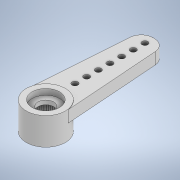
# Autodesk Inventor part: Серво-насадка односторонняя
Saved by Autodesk Inventor 2020 (Build 240168000, 168)
## iProperties
Created: 2021-04-04
Part Number: Серво-насадка односторонняя
Material: Типовые
Document SubType Name: Modeling
Designer: Антон
Density: 1 g/cm^3
Appearance: По умолчанию
Author: Антон
Autodesk Inventor part; units mm, degrees
ref_plane "YZ Plane" through (0, 0, 0) normal (1, 0, 0) x (0, 1, 0)
ref_plane "XZ Plane" through (0, 0, 0) normal (0, 1, 0) x (-1, 0, 0)
ref_plane "XY Plane" through (0, 0, 0) normal (0, 0, 1) x (1, 0, 0)
sketch "Эскиз1" plane through (0, 0, 0) normal (0, 1, 0) x (-1, 0, 0)
  circle A0 centre (0, 0) radius 3.35
  dimension "d0" = 6.7
  constraints: 1 centre point, 1 coincident
  measures "d0" diameter of A0
extrude "Выдавливание1" add sketch "Эскиз1" along normal blind 4.7
ref_plane "РабПлоскость1" through (0, 4.6, 0) normal (0, 1, 0) x (1, 0, 0)
sketch "Эскиз2" plane through (0, 4.6, 0) normal (0, 1, 0) x (1, 0, 0)
  circle A0 centre (0, 0) radius 3.35 projected
  circle A1 centre (0, 0) radius 3.35 projected
  line L0 (-3.35, 0) -> (3.35, 0)
  line L1 (3.35, 0) -> (3.35, 18.5)
  line L2 (3.35, 18.5) -> (-3.35, 18.5)
  line L3 (-3.35, 18.5) -> (-3.35, 0)
  line L4 (2, 0) -> (2, 18.5)
  line L5 (2, 18.5) -> (-2, 18.5)
  line L6 (-2, 18.5) -> (-2, 0)
  line L7 (-2, 0) -> (2, 0)
  line L8 (2, 0) -> (-2, 18.5) construction
  line L9 (2, 18.5) -> (-2, 0) construction
  line L10 (-3.35, 0) -> (-2, 18.5)
  line L11 (3.35, 0) -> (2, 18.5)
  point P0 (0, 9.25)
  point P1 (-3.3145, 0.4863)
  point P2 (3.3145, 0.4863)
  dimension "d4" = 18.5
  dimension "d5" = 4
  constraints: 24 end point, 4 parallel, 2 midpoint, 2 perpendicular, 1 horizontal, 1 horizontal alignment, 1 other
  measures "d4" distance of L1.end L0.end
  measures "d5" distance of L5.end L4.end
extrude "Выдавливание2" add sketch "Эскиз2" against normal blind 2 contours L10 L6 A0 | A0 L4 L11 | L6 L2 L4 A0
sketch "Эскиз3" plane through (0, 4.6, 0) normal (0, 1, 0) x (1, 0, 0)
  line L0 (-2, 18.5) -> (2, 18.5) projected
  line L1 (0, 18.5) -> (0, 17)
  circle A0 centre (0, 17) radius 0.5
  circle A1 centre (0, 15) radius 0.5
  circle A2 centre (0, 13) radius 0.5
  circle A3 centre (0, 11) radius 0.5
  circle A4 centre (0, 9) radius 0.5
  circle A5 centre (0, 7) radius 0.5
  circle A6 centre (0, 5) radius 0.5
  point P0 (0, 0)
  dimension "d8" = 1.5
  dimension "d9" = 1
  dimension "d12" = 2
  constraints: 7 centre point, 2 end point, 2 vertical, 1 coincident, 1 midpoint, 12 other
  measures "d8" distance of L1.start L1.end
  measures "d9" diameter of A0
  measures "d12" distance of A0.centre A1.centre
extrude "Выдавливание3" cut sketch "Эскиз3" against normal through all
fillet "Сопряжение1" radius 2 2 edges at (-2, 3.6, -18.5) (2, 3.6, -18.5)
sketch "Эскиз5" plane through (0, 4.7, 0) normal (0, 1, 0) x (1, 0, 0)
  point P0 (0, 0)
  point P1 (0, 0)
  constraints: 1 coincident
hole "Отверстие1" at (0, 4.7, 0) direction (0, -1, 0) diameter 2.7 end through all counterbore diameter 4.7 counterbore depth 1
sketch "Эскиз6" plane through (0, 0, 0) normal (0, -1, 0) x (1, 0, 0)
  circle A0 centre (0, 0) radius 1.35 projected
  circle A1 centre (0, 0) radius 3.35 projected
  line L0 (0, 0) -> (-2.375, 0)
  line L1 (-2.375, 0) -> (-2.4726, 0.0976)
  line L2 (-2.4726, 0.0976) -> (-2.4692, 0.1615)
  line L3 (-2.375, 0) -> (-2.4726, -0.0976)
  line L4 (-2.362, -0.2483) -> (-2.4692, -0.1614)
  line L5 (-2.4692, -0.1614) -> (-2.4726, -0.0975)
  line L6 (-2.362, -0.2483) -> (-2.4488, -0.3555)
  line L7 (-2.3231, -0.4938) -> (-2.4388, -0.4186)
  line L8 (-2.4388, -0.4186) -> (-2.4488, -0.3554)
  line L9 (-2.3231, -0.4938) -> (-2.3983, -0.6095)
  line L10 (-2.2588, -0.7339) -> (-2.3817, -0.6713)
  line L11 (-2.3817, -0.6713) -> (-2.3983, -0.6094)
  line L12 (-2.2588, -0.7339) -> (-2.3214, -0.8569)
  line L13 (-2.1697, -0.966) -> (-2.2985, -0.9165)
  line L14 (-2.2985, -0.9165) -> (-2.3214, -0.8568)
  line L15 (-2.1697, -0.966) -> (-2.2191, -1.0948)
  line L16 (-2.0568, -1.1875) -> (-2.1901, -1.1518)
  line L17 (-2.1901, -1.1518) -> (-2.2192, -1.0948)
  line L18 (-2.0568, -1.1875) -> (-2.0925, -1.3208)
  line L19 (-1.9214, -1.396) -> (-2.0577, -1.3744)
  line L20 (-2.0577, -1.3744) -> (-2.0926, -1.3207)
  line L21 (-1.9214, -1.396) -> (-1.943, -1.5323)
  line L22 (-1.765, -1.5892) -> (-1.9028, -1.582)
  line L23 (-1.9028, -1.582) -> (-1.9431, -1.5322)
  line L24 (-1.765, -1.5892) -> (-1.7722, -1.727)
  line L25 (-1.5892, -1.765) -> (-1.727, -1.7722)
  line L26 (-1.727, -1.7722) -> (-1.7723, -1.7269)
  line L27 (-1.5892, -1.765) -> (-1.582, -1.9028)
  line L28 (-1.396, -1.9214) -> (-1.5323, -1.943)
  line L29 (-1.5323, -1.943) -> (-1.582, -1.9027)
  line L30 (-1.396, -1.9214) -> (-1.3744, -2.0577)
  line L31 (-1.1875, -2.0568) -> (-1.3208, -2.0925)
  line L32 (-1.3208, -2.0925) -> (-1.3745, -2.0577)
  line L33 (-1.1875, -2.0568) -> (-1.1518, -2.1901)
  line L34 (-0.966, -2.1697) -> (-1.0948, -2.2191)
  line L35 (-1.0948, -2.2191) -> (-1.1519, -2.1901)
  line L36 (-0.966, -2.1697) -> (-0.9165, -2.2985)
  line L37 (-0.7339, -2.2588) -> (-0.8569, -2.3214)
  line L38 (-0.8569, -2.3214) -> (-0.9166, -2.2985)
  line L39 (-0.7339, -2.2588) -> (-0.6713, -2.3817)
  line L40 (-0.4938, -2.3231) -> (-0.6095, -2.3983)
  line L41 (-0.6095, -2.3983) -> (-0.6713, -2.3817)
  line L42 (-0.4938, -2.3231) -> (-0.4186, -2.4388)
  line L43 (-0.2483, -2.362) -> (-0.3555, -2.4488)
  line L44 (-0.3555, -2.4488) -> (-0.4187, -2.4388)
  line L45 (-0.2483, -2.362) -> (-0.1614, -2.4692)
  line L46 (0, -2.375) -> (-0.0976, -2.4726)
  line L47 (-0.0976, -2.4726) -> (-0.1615, -2.4692)
  line L48 (0, -2.375) -> (0.0976, -2.4726)
  line L49 (0.2483, -2.362) -> (0.1614, -2.4692)
  line L50 (0.1614, -2.4692) -> (0.0975, -2.4726)
  line L51 (0.2483, -2.362) -> (0.3555, -2.4488)
  line L52 (0.4938, -2.3231) -> (0.4186, -2.4388)
  line L53 (0.4186, -2.4388) -> (0.3554, -2.4488)
  line L54 (0.4938, -2.3231) -> (0.6095, -2.3983)
  line L55 (0.7339, -2.2588) -> (0.6713, -2.3817)
  line L56 (0.6713, -2.3817) -> (0.6094, -2.3983)
  line L57 (0.7339, -2.2588) -> (0.8569, -2.3214)
  line L58 (0.966, -2.1697) -> (0.9165, -2.2985)
  line L59 (0.9165, -2.2985) -> (0.8568, -2.3214)
  line L60 (0.966, -2.1697) -> (1.0948, -2.2191)
  line L61 (1.1875, -2.0568) -> (1.1518, -2.1901)
  line L62 (1.1518, -2.1901) -> (1.0948, -2.2192)
  line L63 (1.1875, -2.0568) -> (1.3208, -2.0925)
  line L64 (1.396, -1.9214) -> (1.3744, -2.0577)
  line L65 (1.3744, -2.0577) -> (1.3207, -2.0926)
  line L66 (1.396, -1.9214) -> (1.5323, -1.943)
  line L67 (1.5892, -1.765) -> (1.582, -1.9028)
  line L68 (1.582, -1.9028) -> (1.5322, -1.9431)
  line L69 (1.5892, -1.765) -> (1.727, -1.7722)
  line L70 (1.765, -1.5892) -> (1.7722, -1.727)
  line L71 (1.7722, -1.727) -> (1.7269, -1.7723)
  line L72 (1.765, -1.5892) -> (1.9028, -1.582)
  line L73 (1.9214, -1.396) -> (1.943, -1.5323)
  line L74 (1.943, -1.5323) -> (1.9027, -1.582)
  line L75 (1.9214, -1.396) -> (2.0577, -1.3744)
  line L76 (2.0568, -1.1875) -> (2.0925, -1.3208)
  line L77 (2.0925, -1.3208) -> (2.0577, -1.3745)
  line L78 (2.0568, -1.1875) -> (2.1901, -1.1518)
  line L79 (2.1697, -0.966) -> (2.2191, -1.0948)
  line L80 (2.2191, -1.0948) -> (2.1901, -1.1519)
  line L81 (2.1697, -0.966) -> (2.2985, -0.9165)
  line L82 (2.2588, -0.7339) -> (2.3214, -0.8569)
  line L83 (2.3214, -0.8569) -> (2.2985, -0.9166)
  line L84 (2.2588, -0.7339) -> (2.3817, -0.6713)
  line L85 (2.3231, -0.4938) -> (2.3983, -0.6095)
  line L86 (2.3983, -0.6095) -> (2.3817, -0.6713)
  line L87 (2.3231, -0.4938) -> (2.4388, -0.4186)
  line L88 (2.362, -0.2483) -> (2.4488, -0.3555)
  line L89 (2.4488, -0.3555) -> (2.4388, -0.4187)
  line L90 (2.362, -0.2483) -> (2.4692, -0.1614)
  line L91 (2.375, 0) -> (2.4726, -0.0976)
  line L92 (2.4726, -0.0976) -> (2.4692, -0.1615)
  line L93 (2.375, 0) -> (2.4726, 0.0976)
  line L94 (2.362, 0.2483) -> (2.4692, 0.1614)
  line L95 (2.4692, 0.1614) -> (2.4726, 0.0975)
  line L96 (2.362, 0.2483) -> (2.4488, 0.3555)
  line L97 (2.3231, 0.4938) -> (2.4388, 0.4186)
  line L98 (2.4388, 0.4186) -> (2.4488, 0.3554)
  line L99 (2.3231, 0.4938) -> (2.3983, 0.6095)
  line L100 (2.2588, 0.7339) -> (2.3817, 0.6713)
  line L101 (2.3817, 0.6713) -> (2.3983, 0.6094)
  line L102 (2.2588, 0.7339) -> (2.3214, 0.8569)
  line L103 (2.1697, 0.966) -> (2.2985, 0.9165)
  line L104 (2.2985, 0.9165) -> (2.3214, 0.8568)
  line L105 (2.1697, 0.966) -> (2.2191, 1.0948)
  line L106 (2.0568, 1.1875) -> (2.1901, 1.1518)
  line L107 (2.1901, 1.1518) -> (2.2192, 1.0948)
  line L108 (2.0568, 1.1875) -> (2.0925, 1.3208)
  line L109 (1.9214, 1.396) -> (2.0577, 1.3744)
  line L110 (2.0577, 1.3744) -> (2.0926, 1.3207)
  line L111 (1.9214, 1.396) -> (1.943, 1.5323)
  line L112 (1.765, 1.5892) -> (1.9028, 1.582)
  line L113 (1.9028, 1.582) -> (1.9431, 1.5322)
  line L114 (1.765, 1.5892) -> (1.7722, 1.727)
  line L115 (1.5892, 1.765) -> (1.727, 1.7722)
  line L116 (1.727, 1.7722) -> (1.7723, 1.7269)
  line L117 (1.5892, 1.765) -> (1.582, 1.9028)
  line L118 (1.396, 1.9214) -> (1.5323, 1.943)
  line L119 (1.5323, 1.943) -> (1.582, 1.9027)
  line L120 (1.396, 1.9214) -> (1.3744, 2.0577)
  line L121 (1.1875, 2.0568) -> (1.3208, 2.0925)
  line L122 (1.3208, 2.0925) -> (1.3745, 2.0577)
  line L123 (1.1875, 2.0568) -> (1.1518, 2.1901)
  line L124 (0.966, 2.1697) -> (1.0948, 2.2191)
  line L125 (1.0948, 2.2191) -> (1.1519, 2.1901)
  line L126 (0.966, 2.1697) -> (0.9165, 2.2985)
  line L127 (0.7339, 2.2588) -> (0.8569, 2.3214)
  line L128 (0.8569, 2.3214) -> (0.9166, 2.2985)
  line L129 (0.7339, 2.2588) -> (0.6713, 2.3817)
  line L130 (0.4938, 2.3231) -> (0.6095, 2.3983)
  line L131 (0.6095, 2.3983) -> (0.6713, 2.3817)
  line L132 (0.4938, 2.3231) -> (0.4186, 2.4388)
  line L133 (0.2483, 2.362) -> (0.3555, 2.4488)
  line L134 (0.3555, 2.4488) -> (0.4187, 2.4388)
  line L135 (0.2483, 2.362) -> (0.1614, 2.4692)
  line L136 (0, 2.375) -> (0.0976, 2.4726)
  line L137 (0.0976, 2.4726) -> (0.1615, 2.4692)
  line L138 (0, 2.375) -> (-0.0976, 2.4726)
  line L139 (-0.2483, 2.362) -> (-0.1614, 2.4692)
  line L140 (-0.1614, 2.4692) -> (-0.0975, 2.4726)
  line L141 (-0.2483, 2.362) -> (-0.3555, 2.4488)
  line L142 (-0.4938, 2.3231) -> (-0.4186, 2.4388)
  line L143 (-0.4186, 2.4388) -> (-0.3554, 2.4488)
  line L144 (-0.4938, 2.3231) -> (-0.6095, 2.3983)
  line L145 (-0.7339, 2.2588) -> (-0.6713, 2.3817)
  line L146 (-0.6713, 2.3817) -> (-0.6094, 2.3983)
  line L147 (-0.7339, 2.2588) -> (-0.8569, 2.3214)
  line L148 (-0.966, 2.1697) -> (-0.9165, 2.2985)
  line L149 (-0.9165, 2.2985) -> (-0.8568, 2.3214)
  line L150 (-0.966, 2.1697) -> (-1.0948, 2.2191)
  line L151 (-1.1875, 2.0568) -> (-1.1518, 2.1901)
  line L152 (-1.1518, 2.1901) -> (-1.0948, 2.2192)
  line L153 (-1.1875, 2.0568) -> (-1.3208, 2.0925)
  line L154 (-1.396, 1.9214) -> (-1.3744, 2.0577)
  line L155 (-1.3744, 2.0577) -> (-1.3207, 2.0926)
  line L156 (-1.396, 1.9214) -> (-1.5323, 1.943)
  line L157 (-1.5892, 1.765) -> (-1.582, 1.9028)
  line L158 (-1.582, 1.9028) -> (-1.5322, 1.9431)
  line L159 (-1.5892, 1.765) -> (-1.727, 1.7722)
  line L160 (-1.765, 1.5892) -> (-1.7722, 1.727)
  line L161 (-1.7722, 1.727) -> (-1.7269, 1.7723)
  line L162 (-1.765, 1.5892) -> (-1.9028, 1.582)
  line L163 (-1.9214, 1.396) -> (-1.943, 1.5323)
  line L164 (-1.943, 1.5323) -> (-1.9027, 1.582)
  line L165 (-1.9214, 1.396) -> (-2.0577, 1.3744)
  line L166 (-2.0568, 1.1875) -> (-2.0925, 1.3208)
  line L167 (-2.0925, 1.3208) -> (-2.0577, 1.3745)
  line L168 (-2.0568, 1.1875) -> (-2.1901, 1.1518)
  line L169 (-2.1697, 0.966) -> (-2.2191, 1.0948)
  line L170 (-2.2191, 1.0948) -> (-2.1901, 1.1519)
  line L171 (-2.1697, 0.966) -> (-2.2985, 0.9165)
  line L172 (-2.2588, 0.7339) -> (-2.3214, 0.8569)
  line L173 (-2.3214, 0.8569) -> (-2.2985, 0.9166)
  line L174 (-2.2588, 0.7339) -> (-2.3817, 0.6713)
  line L175 (-2.3231, 0.4938) -> (-2.3983, 0.6095)
  line L176 (-2.3983, 0.6095) -> (-2.3817, 0.6713)
  line L177 (-2.3231, 0.4938) -> (-2.4388, 0.4186)
  line L178 (-2.362, 0.2483) -> (-2.4488, 0.3555)
  line L179 (-2.4488, 0.3555) -> (-2.4388, 0.4187)
  line L180 (-2.362, 0.2483) -> (-2.4692, 0.1614)
  dimension "d30" = 2.375
  dimension "d31" = 0.138
  dimension "d32" = 135
  dimension "d34" = 0.064
  dimension "d35" = 132
  dimension "d36" = 0.138
  dimension "d37" = 135
  dimension "d40" = 360
  constraints: 362 end point, 1 horizontal, 421 other
  measures "d30" distance of L0.start L0.end
  measures "d31" distance of L0.end L1.end
  measures "d32" angle of L0 L1
  measures "d34" distance of L1.end L2.end
  measures "d35" angle of L1 L2
  measures "d36" distance of L0.end L3.end
  measures "d37" angle of L0 L3
extrude "Выдавливание5" cut sketch "Эскиз6" against normal blind 3 contours L1 L2 L180 L178 L179 L177 L175 L176 L174 L172 L173 L171 L169 L170 L168 L166 L167 L165 L163 L164 L162 L160 L161 L159 L157 L158 L156 L154 L155 L153 L151 L152 L150 L148 L149 L147 L145 L146 L144 L142 L143 L141 L139 L140 L138 L136 L137 L135 L133 L134 L132 L130 L131 L129 L127 L128 L126 L124 L125 L123 L121 L122 L120 L118 L119 L117 L115 L116 L114 L112 L113 L111 L109 L110 L108 L106 L107 L105 L103 L104 L102 L100 L101 L99 L97 L98 L96 L94 L95 L93 L91 L92 L90 L88 L89 L87 L85 L86 L84 L82 L83 L81 L79 L80 L78 L76 L77 L75 L73 L74 L72 L70 L71 L69 L67 L68 L66 L64 L65 L63 L61 L62 L60 L58 L59 L57 L55 L56 L54 L52 L53 L51 L49 L50 L48 L46 L47 L45 L43 L44 L42 L40 L41 L39 L37 L38 L36 L34 L35 L33 L31 L32 L30 L28 L29 L27 L25 L26 L24 L22 L23 L21 L19 L20 L18 L16 L17 L15 L13 L14 L12 L10 L11 L9 L7 L8 L6 L4 L5 L3
equation "\"d12\" = d8 + 0.5 * d9"
